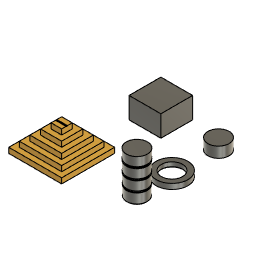
printer calibration v6 (Autodesk Fusion 360 design; units mm, degrees)
Autodesk Fusion 360 part; units mm, degrees
note: some values were not read from the file. Set by a fixed rule: which face or edge a step refers to.
sketch "Sketch1" plane through (0, 0, 0) normal (0, 0, 1) x (1, 0, 0) in component "size test"
  line L0 (25, -25) -> (-25, -25)
  line L1 (-25, -25) -> (-25, 25)
  line L2 (-25, 25) -> (25, 25)
  line L3 (25, 25) -> (25, -25)
  line L4 (25, -25) -> (-25, 25) construction
  line L5 (-25, -25) -> (25, 25) construction
  line L6 (20, -20) -> (-20, -20)
  line L7 (-20, -20) -> (-20, 20)
  line L8 (-20, 20) -> (20, 20)
  line L9 (20, 20) -> (20, -20)
  line L10 (20, -20) -> (-20, 20) construction
  line L11 (-20, -20) -> (20, 20) construction
  line L12 (15, -15) -> (-15, -15)
  line L13 (-15, -15) -> (-15, 15)
  line L14 (-15, 15) -> (15, 15)
  line L15 (15, 15) -> (15, -15)
  line L16 (15, -15) -> (-15, 15) construction
  line L17 (-15, -15) -> (15, 15) construction
  line L18 (10, -10) -> (-10, -10)
  line L19 (-10, -10) -> (-10, 10)
  line L20 (-10, 10) -> (10, 10)
  line L21 (10, 10) -> (10, -10)
  line L22 (10, -10) -> (-10, 10) construction
  line L23 (-10, -10) -> (10, 10) construction
  line L24 (5, -5) -> (-5, -5)
  line L25 (-5, -5) -> (-5, 5)
  line L26 (-5, 5) -> (5, 5)
  line L27 (5, 5) -> (5, -5)
  line L28 (5, -5) -> (-5, 5) construction
  line L29 (-5, -5) -> (5, 5) construction
  dimension "d33" = 50
  dimension "d34" = 50
  dimension "d35" = 40
  dimension "d36" = 40
  dimension "d37" = 30
  dimension "d38" = 30
  dimension "d39" = 20
  dimension "d40" = 20
  dimension "d41" = 10
  dimension "d42" = 10
  constraint horizontal L0
  constraint perpendicular L0 L1
  constraint parallel L0 L2
  constraint parallel L1 L3
  constraint coincident L4 origin
  constraint coincident L5 origin
  constraint horizontal L6
  constraint perpendicular L6 L7
  constraint parallel L6 L8
  constraint parallel L7 L9
  constraint coincident L10 origin
  constraint coincident L11 origin
  constraint horizontal L12
  constraint perpendicular L12 L13
  constraint parallel L12 L14
  constraint parallel L13 L15
  constraint coincident L16 origin
  constraint coincident L17 origin
  constraint horizontal L18
  constraint perpendicular L18 L19
  constraint parallel L18 L20
  constraint parallel L19 L21
  constraint coincident L22 origin
  constraint coincident L23 origin
  constraint horizontal L24
  constraint perpendicular L24 L25
  constraint parallel L24 L26
  constraint parallel L25 L27
  constraint coincident L28 origin
  constraint coincident L29 origin
  measures "d33" distance of L1.end L2.end
  measures "d34" distance of L0.end L1.end
  measures "d35" distance of L7.end L8.end
  measures "d36" distance of L6.end L7.end
  measures "d37" distance of L13.end L14.end
  measures "d38" distance of L12.end L13.end
  measures "d39" distance of L19.end L20.end
  measures "d40" distance of L18.end L19.end
  measures "d41" distance of L25.end L26.end
  measures "d42" distance of L24.end L25.end
extrude "Extrude2" add sketch "Sketch1" along normal blind 25 contours L24 L25 L26 L27 makes body 1 in component "size test"
extrude "Extrude3" add sketch "Sketch1" along normal blind 20 contours L18 L19 L20 L21 bodies 1 in component "size test"
extrude "Extrude4" add sketch "Sketch1" along normal blind 15 contours L12 L13 L14 L15 bodies 1 in component "size test"
extrude "Extrude5" add sketch "Sketch1" along normal blind 10 contours L6 L7 L8 L9 bodies 1 in component "size test"
extrude "Extrude6" add sketch "Sketch1" along normal blind 5 contours L0 L1 L2 L3 bodies 1 in component "size test"
sketch "Sketch1 (2)" plane through (0, 0, 0) normal (0, 0, 1) x (1, 0, 0) in component "seam test"
  circle A0 centre (0, 0) radius 10
  dimension "d26" = 20
  constraint coincident A0.centre origin
  measures "d26" diameter of A0
extrude "Extrude1" add sketch "Sketch1 (2)" along normal blind 10 separate body makes body 2 in component "seam test"
sketch "Sketch2" plane through (0, 0, 0) normal (0, 0, 1) x (1, 0, 0) in component "Flow test"
  line L0 (15, -15) -> (-15, -15)
  line L1 (-15, -15) -> (-15, 15)
  line L2 (-15, 15) -> (15, 15)
  line L3 (15, 15) -> (15, -15)
  line L4 (15, -15) -> (-15, 15) construction
  line L5 (-15, -15) -> (15, 15) construction
  dimension "d29" = 30
  dimension "d30" = 30
  constraint horizontal L0
  constraint perpendicular L0 L1
  constraint parallel L0 L2
  constraint parallel L1 L3
  constraint coincident L4 origin
  constraint coincident L5 origin
  measures "d29" distance of L1.end L2.end
  measures "d30" distance of L0.end L1.end
extrude "Extrude3'" add sketch "Sketch2" along normal blind 20 separate body makes body 3 in component "Flow test"
sketch "Sketch2 (2)" plane through (0, 0, 25) normal (0, 0, 1) x (-1, 0, 0) in component "size test"
  line L0 (-5, -5) -> (5, -5)
  line L1 (5, -5) -> (5, 5)
  line L2 (5, 5) -> (-5, 5)
  line L3 (-5, 5) -> (-5, -5)
  line L4 (5, 0.5) -> (-5, 0.5)
  line L5 (-5, 0.5) -> (-5, -0.5)
  line L6 (-5, -0.5) -> (5, -0.5)
  line L7 (5, -0.5) -> (5, 0.5)
  line L8 (5, 0.5) -> (-5, -0.5) construction
  line L9 (-5, 0.5) -> (5, -0.5) construction
  dimension "d43" = 1
  constraint horizontal L4
  constraint perpendicular L4 L5
  constraint parallel L4 L6
  constraint parallel L5 L7
  constraint coincident L8 origin
  constraint coincident L9 origin
  measures "d43" distance of L4.end L5.end
extrude "Extrude7" cut sketch "Sketch2 (2)" against normal blind 0.3 contours L1 L3 L4 L5 L6 L7 bodies 1 in component "size test"
sketch "Sketch1 (3)" plane through (0, 0, 0) normal (0, 0, 1) x (1, 0, 0) in component "Hole calibration"
  circle A0 centre (0, 0) radius 10
  circle A1 centre (0, 0) radius 15
  circle A2 centre (0, 0) radius 9
  dimension "d46" = 20
  dimension "d47" = 30
  dimension "d59" = 18
  constraint coincident A0.centre A1.centre
  measures "d46" diameter of A0
  measures "d47" diameter of A1
  measures "d59" diameter of A2
extrude "Extrude1'" add sketch "Sketch1 (3)" along normal blind 40 separate body contours A0 | A2 makes body 4 in component "Hole calibration"
extrude "Extrude7'" cut sketch "Sketch1 (3)" along normal blind 1 from surface at 30 contours A0 bodies 4 in component "Hole calibration"
extrude "Extrude8" cut sketch "Sketch1 (3)" along normal blind 1 from surface at 10 contours A0 bodies 4 in component "Hole calibration"
extrude "Extrude9" cut sketch "Sketch1 (3)" along normal blind 1 from surface at 20 contours A0 bodies 4 in component "Hole calibration"
chamfer "Chamfer2" distance 0.7 angle 45 3 edges at (-9.3233, -3.6162, 11) (-9.3233, -3.6162, 21) (-9.3233, -3.6162, 31) on bodies 4 in component "Hole calibration"
extrude "Extrude10" add sketch "Sketch1 (3)" along normal blind 5 separate body contours A1 makes body 5 in component "Hole calibration"
move_body "Move1" bodies 5 to x (1, 0, 0) y (0, 1, 0) z (0, 0, 1) at (0, 33.1761, 0) in component "Hole calibration"
chamfer "Chamfer3" distance 1 angle 45 2 edges at (-9.3233, 36.7922, 0) (-9.3233, -3.6162, 0) on bodies 4 5 in component "Hole calibration"
move_face "OffsetFaces4" offset -0.1 1 faces at (9.9503, -0.9957, 27.2333) on bodies 4 in component "Hole calibration"
move_face "OffsetFaces5" offset -0.2 1 faces at (9.9503, 0.9957, 14.4667) on bodies 4 in component "Hole calibration"
move_face "OffsetFaces6" offset -0.3 1 faces at (9.9503, 0.9957, 4) on bodies 4 in component "Hole calibration"
component "Flow test" placed x (1, 0, 0) y (0, 1, 0) z (0, 0, 1) at (-51.6608, 74.28, 0)
component "size test" placed x (1, 0, 0) y (0, 1, 0) z (0, 0, 1) at (-71.1077, 0, 0)
component "seam test" placed x (1, 0, 0) y (0, 1, 0) z (0, 0, 1) at (0, 77.1099, 0)
component "Hole calibration" placed x (1, 0, 0) y (0, 1, 0) z (0, 0, 1) at (0, 0, 0)
